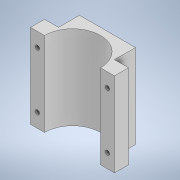
# Autodesk Inventor part: boltSideForclampForMeadeTripodLeg
Saved by Autodesk Inventor 2021.2 (Build 252289000, 289)
## iProperties
Created: 2021-02-07
Part Number: boltSideForclampForMeadeTripodLeg
Material: Generic
Document SubType Name: Modeling
Designer: robst
Density: 1 g/cm^3
Appearance: Default
Author: robst
Autodesk Inventor part; units mm, degrees
ref_plane "YZ Plane" through (0, 0, 0) normal (1, 0, 0) x (0, 1, 0)
ref_plane "XZ Plane" through (0, 0, 0) normal (0, 1, 0) x (-1, 0, 0)
ref_plane "XY Plane" through (0, 0, 0) normal (0, 0, 1) x (1, 0, 0)
sketch "Sketch18" plane through (0, 0, 0) normal (0, 1, 0) x (-1, 0, 0)
  arc A0 (-25.4, 0) -> (25.4, 0) centre (0, 0) ccw
  line L0 (-38.1, 0) -> (-38.1, -31.75)
  line L1 (-38.1, -31.75) -> (38.1, -31.75)
  line L2 (38.1, -31.75) -> (38.1, 0)
  line L3 (38.1, 31.75) -> (-38.1, -31.75) construction
  line L4 (-38.1, 31.75) -> (38.1, -31.75) construction
  line L5 (38.1, 0) -> (25.4, 0)
  line L6 (-25.4, 0) -> (-38.1, 0)
  dimension "d78" = 50.8
  dimension "d79" = 6.35
  dimension "d80" = 12.7
  constraints: 14 end point, 2 midpoint, 2 point on circle, 1 centre point, 1 coincident, 1 parallel
  measures "d78" diameter of A0
  measures "d79" distance edge to line of A0 L1
  measures "d80" distance edge to line of A0 L2
extrude "Extrusion9" add sketch "Sketch18" against normal blind 76.2
sketch "Sketch19" plane through (-38.1, 0, 0) normal (0, 0, 1) x (1, 0, 0)
  line L0 (0, 0) -> (0, -76.2) projected
  line L1 (12.7, 0) -> (12.7, -76.2) projected
  line L2 (63.5, 0) -> (63.5, -76.2) projected
  line L3 (76.2, 0) -> (76.2, -76.2) projected
  line L4 (76.2, -76.2) -> (63.5, -76.2) projected
  line L5 (12.7, -76.2) -> (0, -76.2) projected
  line L6 (0, 0) -> (12.7, 0) projected
  line L7 (63.5, 0) -> (76.2, 0) projected
  line L8 (6.35, -63.5) -> (69.85, -63.5) construction
  line L9 (69.85, -63.5) -> (69.85, -12.7) construction
  line L10 (69.85, -12.7) -> (6.35, -12.7) construction
  line L11 (6.35, -12.7) -> (6.35, -63.5) construction
  line L12 (63.5, -76.2) -> (12.7, -76.2) construction
  line L13 (12.7, 0) -> (63.5, 0) construction
  point P0 (38.1, 0)
  dimension "d83" = 6.35
  dimension "d84" = 6.35
  dimension "d85" = 12.7
  dimension "d86" = 12.7
  constraints: 8 end point, 4 coincident, 2 parallel, 1 horizontal, 1 perpendicular
  measures "d83" distance between parallel lines of L11 L0
  measures "d84" distance between parallel lines of L9 L3
  measures "d85" distance between parallel lines of L12 L8
  measures "d86" distance between parallel lines of L10 L13
hole "Hole3" at (-31.75, -12.7, 0) at (31.75, -12.7, 0) at (31.75, -63.5, 0) at (-31.75, -63.5, 0) direction (0, 0, -1) diameter 3.81 end through all clearance for "Flat Head Machine Screw (82)" size "#6" standard "Ansi Unified Screw Threads"
sketch "Sketch20" plane through (38.1, 0, -31.75) normal (0, 0, -1) x (-1, 0, 0)
  line L0 (76.2, 0) -> (76.2, -76.2) projected
  line L1 (0, 0) -> (76.2, 0) projected
  line L2 (0, 0) -> (0, -76.2) projected
  line L3 (76.2, -76.2) -> (0, -76.2) projected
  line L4 (25.4, -63.5) -> (50.8, -63.5) construction
  line L5 (50.8, -63.5) -> (50.8, -12.7) construction
  line L6 (50.8, -12.7) -> (25.4, -12.7) construction
  line L7 (25.4, -12.7) -> (25.4, -63.5) construction
  line L8 (25.4, -63.5) -> (50.8, -12.7) construction
  line L9 (50.8, -63.5) -> (25.4, -12.7) construction
  line L10 (0, 0) -> (0, -76.2) construction
  point P0 (38.1, 0)
  point P1 (38.1, -38.1)
  dimension "d94" = 12.7
  dimension "d95" = 12.7
  dimension "d96" = 25.4
  dimension "d97" = 25.4
  constraints: 12 end point, 4 coincident, 2 midpoint, 2 parallel, 2 perpendicular
  measures "d94" distance between parallel lines of L6 L1
  measures "d95" distance between parallel lines of L4 L3
  measures "d96" distance between parallel lines of L2 L7
  measures "d97" distance between parallel lines of L0 L5
hole "Hole4" at (12.7, -12.7, -31.75) at (-12.7, -12.7, -31.75) at (-12.7, -63.5, -31.75) at (12.7, -63.5, -31.75) direction (0, 0, 1) diameter 4.7244 depth 7.1501 counterbore diameter 5.1816 counterbore depth 5.5626
sketch "Sketch21" plane through (0, 0, 0) normal (0, 1, 0) x (1, 0, 0)
  line L0 (38.1, 31.75) -> (-38.1, 31.75) projected
  arc A0 (25.4, 0) -> (-25.4, 0) centre (0, 0) ccw projected
  line L1 (38.1, 0) -> (38.1, 31.75) projected
  line L2 (-38.1, 31.75) -> (-38.1, 0) projected
  line L3 (-38.1, 0) -> (-25.4, 0) projected
  line L4 (25.4, 0) -> (38.1, 0) projected
  line L5 (-38.1, 31.75) -> (38.1, 31.75) projected
  line L6 (-38.1, 31.75) -> (-25.4, 31.75)
  line L7 (-25.4, 31.75) -> (-25.4, 12.7)
  line L8 (-25.4, 12.7) -> (-38.1, 12.7)
  line L9 (-38.1, 12.7) -> (-38.1, 31.75)
  line L10 (38.1, 31.75) -> (25.4, 31.75)
  line L11 (25.4, 31.75) -> (25.4, 12.7)
  line L12 (25.4, 12.7) -> (38.1, 12.7)
  line L13 (38.1, 12.7) -> (38.1, 31.75)
  dimension "d105" = 19.05
  dimension "d106" = 12.7
  dimension "d107" = 19.05
  constraints: 16 end point, 4 parallel, 2 horizontal, 2 perpendicular
  measures "d105" distance of L6.end L7.end
  measures "d106" distance between parallel lines of L11 L1
  measures "d107" distance between parallel lines of L0 L12
extrude "Extrusion10" cut sketch "Sketch21" against normal through all contours L1 L12 L11 L0 | L7 L8 L2 L0
equation "\"d78\" = legDiameter"
equation "\"d81\" = legPartHeight"
equation "\"d98\" = diameterOfBottomOfHeatInsert"
equation "\"d100\" = diameterOfTopOfHeatInsert"
equation "\"d101\" = heightOfTopOfHeatInsert"
equation "\"d103\" = heightOfBottomOfHeatInsert"
equation "\"legDiameter\" = 50.8"
equation "\"legWalThickness\" = 3.175"
equation "\"legPartHeight\" = 76.2"
equation "\"heightOfBottomOfHeatInsert\" = 1.5875"
equation "\"heightOfTopOfHeatInsert\" = 5.5626"
equation "\"diameterOfBottomOfHeatInsert\" = 4.7244"
equation "\"diameterOfTopOfHeatInsert\" = 5.1816"
body "Solid1"
body "Solid2"
